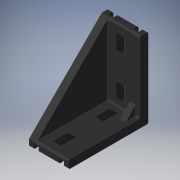
# Autodesk Inventor part: 14070_m
Saved by Autodesk Inventor 2019 (Build 230136000, 136)
## iProperties
Created: 2023-03-27
Part Number: 14070_m
Material: Generic
Catalog Web Link: www.cadenas.de
Description: 14068, 14070, 14080, 14081, 14086, 14088_m-4 Hole Inside Corner Bracket
Vendor: 8020
Document SubType Name: Modeling
Designer: psAdmin
Manufacturer: 8020
Mass: 22.1138 g
Surface Area: 106.342 cm^2
Volume: 22.1138 cm^3
Density: 1 g/cm^3
Appearance: PSOLRGB-175-175-175
Category: PARTsolutions
Company: 8020
Title: 14070
Author: Cadenas PARTsolutions
Comments: 4 Hole Inside Corner Bracket
PSOL_IDENT_0: {$CADENAS_DATA/23d-libs/8020/metric/joining_plates/14068_m.prj},189 {VTYP=3D},{NB=14070_m},{LINA=140
PSOL_IDENT_1: 70},{NN=14068, 14070, 14080, 14081, 14086, 14088_m},{DATE=31.07.2020 09:21:28},{GEOMDATE=09.09.2015
PSOL_IDENT_2: 07:48:54},{VERSION=},{LINEID=10},{WBVAR=D},{WBNUMERIC=}  {NB=14070_m},{LINA=14070},{KT=DUMMY},{PN=14
PSOL_IDENT_3: 070},{MAT=Die Cast Aluminum},{FIN=Natural},{A=57.00},{B=28.00},{C=6.20},{D=8},{D1= '','None','8','8.
PSOL_IDENT_4: 00' },{D2=8.00},{W=.058},{CC=8-30},{NO=1}
NB: 14070_m
NN: 14068, 14070, 14080, 14081, 14086, 14088_m
NT: 4 Hole Inside Corner Bracket
NBSYN: $PN._m
LINA: 14070
CATALOG: 80/20
PN: 14070
MAT: Die Cast Aluminum
FIN: Natural
A: 57
B: 28
C: 6.2
D: 8.00
W: .058
CC: 8-30
SUPPLIER: 8020
ARTICLENO: 14070_m
BOMINFO: 14070
CREATOR: CADENAS GmbH
Autodesk Inventor part; units mm, degrees
ref_plane "YZ Plane" through (0, 0, 0) normal (1, 0, 0) x (0, 1, 0)
ref_plane "XZ Plane" through (0, 0, 0) normal (0, 1, 0) x (-1, 0, 0)
ref_plane "XY Plane" through (0, 0, 0) normal (0, 0, 1) x (1, 0, 0)
sketch "Sketch_1" plane through (0, 0, 0) normal (1, 0, 0) x (0, 1, 0)
  line L0 (1, 57) -> (0, 56)
  line L1 (0, 56) -> (0, 1)
  arc A0 (0, 1) -> (1, 0) centre (1, 1) ccw
  line L2 (1, 0) -> (56, 0)
  line L3 (56, 0) -> (57, 1)
  line L4 (57, 1) -> (57, 5)
  line L5 (57, 5) -> (5, 57)
  line L6 (5, 57) -> (1, 57)
  constraints: 14 end point, 2 point on circle, 1 centre point
extrude "Extrusion1" add sketch "Sketch_1" along normal mid plane 28
sketch "Sketch_2" plane through (-9, 0, 0) normal (1, 0, 0) x (0, 0, -1)
  line L0 (-56, 6) -> (-7, 6)
  arc A0 (-7, 6) -> (-6, 7) centre (-7, 7) ccw
  line L1 (-6, 7) -> (-6, 56)
  line L2 (-6, 56) -> (-56, 6)
  constraints: 6 end point, 2 point on circle, 1 centre point
extrude "Extrusion2" cut sketch "Sketch_2" along normal blind 23
sketch "Sketch_3" plane through (0, 0, 0) normal (1, 0, 0) x (0, 1, 0)
  line L0 (0, 4.6669) -> (0, 1)
  arc A0 (0, 1) -> (1, 0) centre (1, 1) ccw
  line L1 (1, 0) -> (4.6669, 0)
  line L2 (4.6669, 0) -> (2.687, 1.9799)
  line L3 (2.687, 1.9799) -> (1.9799, 1.2728)
  line L4 (1.9799, 1.2728) -> (1.2728, 1.9799)
  line L5 (1.2728, 1.9799) -> (1.9799, 2.687)
  line L6 (1.9799, 2.687) -> (0, 4.6669)
  constraints: 14 end point, 2 point on circle, 1 centre point
extrude "Extrusion3" cut sketch "Sketch_3" along normal mid plane 12
sketch "Sketch_4" plane through (0, 0, 0) normal (1, 0, 0) x (0, 1, 0)
  line L0 (53.8787, 2.1213) -> (51.7574, 0)
  line L1 (51.7574, 0) -> (56, 0)
  line L2 (56, 0) -> (53.8787, 2.1213)
  constraints: 6 end point
extrude "Extrusion4" cut sketch "Sketch_4" along normal mid plane 12
sketch "Sketch_5" plane through (0, 0, 0) normal (1, 0, 0) x (0, 1, 0)
  line L0 (0, 56) -> (0, 51.7574)
  line L1 (0, 51.7574) -> (2.1213, 53.8787)
  line L2 (2.1213, 53.8787) -> (0, 56)
  constraints: 6 end point
extrude "Extrusion5" cut sketch "Sketch_5" along normal mid plane 12
sketch "Sketch_6" plane through (0, 0, 0) normal (1, 0, 0) x (0, 1, 0)
  line L0 (55.2929, 0.7071) -> (53.313, -1.2728)
  line L1 (53.313, -1.2728) -> (54.0201, -1.9799)
  line L2 (54.0201, -1.9799) -> (56, 0)
  line L3 (56, 0) -> (55.2929, 0.7071)
  constraints: 8 end point
extrude "Extrusion6" add sketch "Sketch_6" along normal mid plane 8
sketch "Sketch22" plane through (0, -2.1213, 2.1213) normal (0, -0.7071, 0.7071) x (1, 0, 0)
  line L0 (-4, 3.3) -> (-4, 0.2)
  line L1 (-4, 0.2) -> (4, 0.2)
  line L2 (4, 0.2) -> (4, 3.3)
  line L3 (4, 3.3) -> (-4, 3.3)
  constraints: 8 end point
extrude "Extrusion7" add sketch "Sketch22" against normal blind 1
sketch "Sketch25" plane through (0, 2.1213, -2.1213) normal (0, 0.7071, -0.7071) x (-1, 0, 0)
  line L0 (-4, 3.3) -> (-4, 0.2)
  line L1 (-4, 0.2) -> (4, 0.2)
  line L2 (4, 0.2) -> (4, 3.3)
  line L3 (4, 3.3) -> (-4, 3.3)
  constraints: 8 end point
extrude "Extrusion8" add sketch "Sketch25" against normal blind 1
sketch "Sketch_7" plane through (0, 0, 0) normal (1, 0, 0) x (0, 1, 0)
  line L0 (0, 56) -> (-1.9799, 54.0201)
  line L1 (-1.9799, 54.0201) -> (-1.2728, 53.313)
  line L2 (-1.2728, 53.313) -> (0.7071, 55.2929)
  line L3 (0.7071, 55.2929) -> (0, 56)
  constraints: 8 end point
extrude "Extrusion9" add sketch "Sketch_7" along normal mid plane 8
sketch "Sketch_8" plane through (-9, 0, 0) normal (1, 0, 0) x (0, 0, -1)
  line L0 (-57, 3.7759) -> (-57, 1)
  line L1 (-57, 1) -> (-56, 0)
  line L2 (-56, 0) -> (-52.5, 0)
  line L3 (-52.5, 0) -> (-57, 3.7759)
  constraints: 8 end point
extrude "Extrusion10" cut sketch "Sketch_8" along normal mid plane 4
sketch "Sketch_9" plane through (-9, 0, 0) normal (1, 0, 0) x (0, 0, -1)
  line L0 (-3.7759, 57) -> (0, 52.5)
  line L1 (0, 52.5) -> (0, 56)
  line L2 (0, 56) -> (-1, 57)
  line L3 (-1, 57) -> (-3.7759, 57)
  constraints: 8 end point
extrude "Extrusion11" cut sketch "Sketch_9" along normal mid plane 4
sketch "Sketch_16" plane through (9, 0, 0) normal (1, 0, 0) x (0, 0, -1)
  line L0 (-13.0711, 6) -> (-7, 6)
  arc A0 (-7, 6) -> (-6, 7) centre (-7, 7) ccw
  line L1 (-6, 7) -> (-6, 13.0711)
  line L2 (-6, 13.0711) -> (-13.0711, 6)
  constraints: 6 end point, 2 point on circle, 1 centre point
extrude "Extrusion12" add sketch "Sketch_16" along normal mid plane 4
sketch "Sketch_10" plane through (9, 0, 0) normal (1, 0, 0) x (0, 0, -1)
  line L0 (-3.7759, 57) -> (0, 52.5)
  line L1 (0, 52.5) -> (0, 56)
  line L2 (0, 56) -> (-1, 57)
  line L3 (-1, 57) -> (-3.7759, 57)
  constraints: 8 end point
extrude "Extrusion13" cut sketch "Sketch_10" along normal mid plane 4
sketch "Sketch_11" plane through (9, 0, 0) normal (1, 0, 0) x (0, 0, -1)
  line L0 (-57, 1) -> (-56, 0)
  line L1 (-56, 0) -> (-52.5, 0)
  line L2 (-52.5, 0) -> (-57, 3.7759)
  line L3 (-57, 3.7759) -> (-57, 1)
  constraints: 8 end point
extrude "Extrusion14" cut sketch "Sketch_11" along normal mid plane 4
sketch "Sketch_12" plane through (0, 0, 0) normal (1, 0, 0) x (0, 1, 0)
  line L0 (21, 6) -> (10.2426, 6)
  line L1 (10.2426, 6) -> (4.4548, 0.2121)
  line L2 (4.4548, 0.2121) -> (4.6669, 0)
  line L3 (4.6669, 0) -> (21, 0)
  line L4 (21, 0) -> (21, 6)
  constraints: 10 end point
extrude "Extrusion15" cut sketch "Sketch_12" along normal mid plane 6.2
sketch "Sketch_13" plane through (0, 0, 0) normal (1, 0, 0) x (0, 1, 0)
  line L0 (0, 21) -> (0, 4.6669)
  line L1 (0, 4.6669) -> (0.2121, 4.4548)
  line L2 (0.2121, 4.4548) -> (6, 10.2426)
  line L3 (6, 10.2426) -> (6, 21)
  line L4 (6, 21) -> (0, 21)
  constraints: 10 end point
extrude "Extrusion16" cut sketch "Sketch_13" along normal mid plane 6.2
sketch "Sketch_14" plane through (0, 0, 0) normal (1, 0, 0) x (0, 1, 0)
  line L0 (40, 6) -> (34, 0)
  line L1 (34, 0) -> (51, 0)
  line L2 (51, 0) -> (51, 6)
  line L3 (51, 6) -> (40, 6)
  constraints: 8 end point
extrude "Extrusion17" cut sketch "Sketch_14" along normal mid plane 6.2
sketch "Sketch_15" plane through (0, 0, 0) normal (1, 0, 0) x (0, 1, 0)
  line L0 (0, 51) -> (0, 34)
  line L1 (0, 34) -> (6, 40)
  line L2 (6, 40) -> (6, 51)
  line L3 (6, 51) -> (0, 51)
  constraints: 8 end point
extrude "Extrusion18" cut sketch "Sketch_15" along normal mid plane 6.2
body "Solid1"
